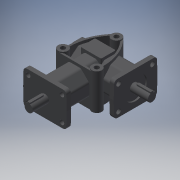
# Autodesk Inventor part: KBX-151L
Saved by Autodesk Inventor 2018 (Build 220112000, 112)
## iProperties
Category: PARTsolutions
Company: KHK
Created: 2017-10-24
Part Number: KBX-151L
Catalog Web Link: www.cadenas.de
Description: Bevel Box (KBXL)-
Vendor: KHK
Document SubType Name: Modeling
Designer: psAdmin
Manufacturer: KHK
Mass: 507.667 g
Surface Area: 746.565 cm^2
Volume: 507.667 cm^3
Density: 1 g/cm^3
Material: 一般
Appearance: PSOLRGB-175-175-175
PSOL_IDENT_0: {$CADENAS_DATA\23d-libs\khk\other_products\bevel_box_kbxl.prj},168 {VTYP=3D},{NB=KBX-151L},{LINA=KBX
PSOL_IDENT_1: -151L},{NN=Bevel Box (KBXL)},{DATE=08.02.2017 09:55:25},{GEOMDATE=11.03.2010 06:12:00},{VERSION=},{L
PSOL_IDENT_2: INEID=40},{LINESUBID=-1},{WBVAR=}  {NB=KBX-151L},{LINA=KBX-151L},{KT=DUMMY},{CN=KBX-151L},{SR=1:1},{
PSOL_IDENT_3: A=66},{B=100},{C=31},{D=36},{E=31},{F=22},{G=80},{H=62},{I=66},{J=140},{K=8},{L=137},{M=170},{P=30},
PSOL_IDENT_4: {Q=8.5},{R=8.5},{S=15},{T=42},{U=3},{KEY=5×5×27L},{WMF=LBX01.WMF},{Q1=8.5},{R1=8.5},{S1=15},{T1=42},
PSOL_IDENT_5: {R11=6},{R12=4.25},{F1=9.5},{F11=5},{F12=27},{E1=52},{E1R=6},{E11=46},{E11R=5},{RGX=57.275},{RGY=73.
PSOL_IDENT_6: 724},{RG1=90},{RG2=86.5},{RG3=9.01},{PLX=38},{PLY=27},{PL=16.23}
NN: Bevel Box (KBXL)
NB: KBX-151L
NBSYN: $CN.
LINA: KBX-151L
CN: KBX-151L
SR: 1:1
A: 66
B: 100
C: 31
D: 36
E: 31
F: 22
G: 80
H: 62
I: 66
J: 140
K: 8
L: 137
M: 170
P: 30
Q: 8.5
R: 8.5
S: 15
T: 42
U: 3
KEY: 5x5x27L
SUPPLIER: KHK
ARTICLENO: KBX-151L
BOMINFO: KBX-151L
CREATOR: CADENAS GmbH
Title: KBX-151L
Author: Cadenas PARTsolutions
Autodesk Inventor part; units mm, degrees
ref_plane "YZ Plane" through (0, 0, 0) normal (1, 0, 0) x (0, 1, 0)
ref_plane "XZ Plane" through (0, 0, 0) normal (0, 1, 0) x (-1, 0, 0)
ref_plane "XY Plane" through (0, 0, 0) normal (0, 0, 1) x (1, 0, 0)
sketch "Sketch_1" plane through (0, 0, 0) normal (0, 1, 0) x (1, 0, 0)
  line L0 (-40, 0) -> (-39.3412, -25.1571)
  arc A0 (-39.3412, -25.1571) -> (-33.3433, -31) centre (-33.3433, -25) ccw
  line L1 (-33.3433, -31) -> (33.3433, -31)
  arc A1 (33.3433, -31) -> (39.3412, -25.1571) centre (33.3433, -25) ccw
  line L2 (39.3412, -25.1571) -> (40, 0)
  line L3 (40, 0) -> (39.3412, 25.1571)
  arc A2 (39.3412, 25.1571) -> (33.3433, 31) centre (33.3433, 25) ccw
  line L4 (33.3433, 31) -> (-33.3433, 31)
  arc A3 (-33.3433, 31) -> (-39.3412, 25.1571) centre (-33.3433, 25) ccw
  line L5 (-39.3412, 25.1571) -> (-40, 0)
  circle A4 centre (31, 22) radius 4.25
  circle A5 centre (31, -22) radius 4.25
  circle A6 centre (-31, 22) radius 4.25
  circle A7 centre (-31, -22) radius 4.25
  constraints: 12 end point, 8 centre point, 8 point on circle
extrude "Extrusion1" add sketch "Sketch_1" along normal blind 8
sketch "Sketch2" plane through (0, 0, 0) normal (0, -1, 0) x (1, 0, 0)
  point P0 (0, 0)
hole "Hole1" at (0, 0, 0) direction (0, 1, 0) diameter 42 depth 3
sketch "Sketch_3" plane through (0, 0, 0) normal (0, 0, 1) x (1, 0, 0)
  line L0 (0, -30) -> (0, 8)
  line L1 (0, 8) -> (7.5, 8)
  line L2 (7.5, 8) -> (7.5, -30)
  line L3 (7.5, -30) -> (0, -30)
  line L4 (0, -30) -> (0, 8)
  constraints: 10 end point
revolve "Revolution1" add sketch "Sketch_3" angle 360 about axis through (0, -30, 0) along (0, -1, 0)
sketch "Sketch_5" plane through (0, 0, 0) normal (0, 0, 1) x (1, 0, 0)
  line L0 (-2.5, -5.5) -> (-2.5, -30)
  line L1 (-2.5, -30) -> (2.5, -30)
  line L2 (2.5, -30) -> (2.5, -5.5)
  arc A0 (2.5, -5.5) -> (-2.5, -5.5) centre (0, -5.5) ccw
  constraints: 6 end point, 2 point on circle, 1 centre point
extrude "Extrusion2" add sketch "Sketch_5" along normal blind 9.5
sketch "Sketch_6" plane through (0, 0, 0) normal (0, 1, 0) x (1, 0, 0)
  line L0 (-26, 8.2843) -> (-26, -8.2843)
  arc A0 (-26, -8.2843) -> (-24.2426, -12.5269) centre (-20, -8.2843) ccw
  line L1 (-24.2426, -12.5269) -> (-12.5269, -24.2426)
  arc A1 (-12.5269, -24.2426) -> (-8.2843, -26) centre (-8.2843, -20) ccw
  line L2 (-8.2843, -26) -> (8.2843, -26)
  arc A2 (8.2843, -26) -> (12.5269, -24.2426) centre (8.2843, -20) ccw
  line L3 (12.5269, -24.2426) -> (24.2426, -12.5269)
  arc A3 (24.2426, -12.5269) -> (26, -8.2843) centre (20, -8.2843) ccw
  line L4 (26, -8.2843) -> (26, 8.2843)
  arc A4 (26, 8.2843) -> (24.2426, 12.5269) centre (20, 8.2843) ccw
  line L5 (24.2426, 12.5269) -> (12.5269, 24.2426)
  arc A5 (12.5269, 24.2426) -> (8.2843, 26) centre (8.2843, 20) ccw
  line L6 (8.2843, 26) -> (-8.2843, 26)
  arc A6 (-8.2843, 26) -> (-12.5269, 24.2426) centre (-8.2843, 20) ccw
  line L7 (-12.5269, 24.2426) -> (-24.2426, 12.5269)
  arc A7 (-24.2426, 12.5269) -> (-26, 8.2843) centre (-20, 8.2843) ccw
  constraints: 16 end point, 16 point on circle, 8 centre point
extrude "Extrusion3" add sketch "Sketch_6" along normal blind 100
sketch "Sketch_7" plane through (0, 0, 0) normal (1, 0, 0) x (0, 0, -1)
  line L0 (-26, 108.2843) -> (-26, 91.7157)
  arc A0 (-26, 91.7157) -> (-24.2426, 87.4731) centre (-20, 91.7157) ccw
  line L1 (-24.2426, 87.4731) -> (-12.5269, 75.7574)
  arc A1 (-12.5269, 75.7574) -> (-8.2843, 74) centre (-8.2843, 80) ccw
  line L2 (-8.2843, 74) -> (8.2843, 74)
  arc A2 (8.2843, 74) -> (12.5269, 75.7574) centre (8.2843, 80) ccw
  line L3 (12.5269, 75.7574) -> (24.2426, 87.4731)
  arc A3 (24.2426, 87.4731) -> (26, 91.7157) centre (20, 91.7157) ccw
  line L4 (26, 91.7157) -> (26, 108.2843)
  arc A4 (26, 108.2843) -> (24.2426, 112.5269) centre (20, 108.2843) ccw
  line L5 (24.2426, 112.5269) -> (12.5269, 124.2426)
  arc A5 (12.5269, 124.2426) -> (8.2843, 126) centre (8.2843, 120) ccw
  line L6 (8.2843, 126) -> (-8.2843, 126)
  arc A6 (-8.2843, 126) -> (-12.5269, 124.2426) centre (-8.2843, 120) ccw
  line L7 (-12.5269, 124.2426) -> (-24.2426, 112.5269)
  arc A7 (-24.2426, 112.5269) -> (-26, 108.2843) centre (-20, 108.2843) ccw
  constraints: 16 end point, 16 point on circle, 8 centre point
extrude "Extrusion4" add sketch "Sketch_7" along normal mid plane 132
sketch "Sketch_9" plane through (0, 0, 0) normal (0, 0, 1) x (1, 0, 0)
  line L0 (-71, 69) -> (-31.5995, 69)
  arc A0 (-10.8459, 131) -> (-31.5995, 69) centre (57.275, 73.724) ccw
  line L1 (-10.8459, 131) -> (-71, 131)
  line L2 (-71, 131) -> (-71, 69)
  constraints: 6 end point, 2 point on circle, 1 centre point
extrude "Extrusion5" cut sketch "Sketch_9" along normal mid plane 80
sketch "Sketch_10" plane through (0, 0, 0) normal (1, 0, 0) x (0, 0, -1)
  line L0 (-23, 107.4558) -> (-23, 92.5442)
  arc A0 (-23, 92.5442) -> (-21.5355, 89.0086) centre (-18, 92.5442) ccw
  line L1 (-21.5355, 89.0086) -> (-10.9914, 78.4645)
  arc A1 (-10.9914, 78.4645) -> (-7.4558, 77) centre (-7.4558, 82) ccw
  line L2 (-7.4558, 77) -> (7.4558, 77)
  arc A2 (7.4558, 77) -> (10.9914, 78.4645) centre (7.4558, 82) ccw
  line L3 (10.9914, 78.4645) -> (21.5355, 89.0086)
  arc A3 (21.5355, 89.0086) -> (23, 92.5442) centre (18, 92.5442) ccw
  line L4 (23, 92.5442) -> (23, 107.4558)
  arc A4 (23, 107.4558) -> (21.5355, 110.9914) centre (18, 107.4558) ccw
  line L5 (21.5355, 110.9914) -> (10.9914, 121.5355)
  arc A5 (10.9914, 121.5355) -> (7.4558, 123) centre (7.4558, 118) ccw
  line L6 (7.4558, 123) -> (-7.4558, 123)
  arc A6 (-7.4558, 123) -> (-10.9914, 121.5355) centre (-7.4558, 118) ccw
  line L7 (-10.9914, 121.5355) -> (-21.5355, 110.9914)
  arc A7 (-21.5355, 110.9914) -> (-23, 107.4558) centre (-18, 107.4558) ccw
  constraints: 16 end point, 16 point on circle, 8 centre point
extrude "Extrusion6" add sketch "Sketch_10" against normal blind 41
sketch "Sketch_11" plane through (0, 0, 0) normal (0, 0, 1) x (1, 0, 0)
  arc A0 (-19, 85.77) -> (-17, 83.77) centre (-17, 85.77) ccw
  line L0 (-17, 83.77) -> (17, 83.77)
  arc A1 (17, 83.77) -> (19, 85.77) centre (17, 85.77) ccw
  line L1 (19, 85.77) -> (19, 108.77)
  arc A2 (19, 108.77) -> (17, 110.77) centre (17, 108.77) ccw
  line L2 (17, 110.77) -> (-17, 110.77)
  arc A3 (-17, 110.77) -> (-19, 108.77) centre (-17, 108.77) ccw
  line L3 (-19, 108.77) -> (-19, 85.77)
  constraints: 8 end point, 8 point on circle, 4 centre point
extrude "Extrusion7" add sketch "Sketch_11" along normal blind 31
sketch "Sketch_12" plane through (0, 0, 0) normal (0, 0, 1) x (1, 0, 0)
  arc A0 (-32.7207, 72.8442) -> (-31, 54.99) centre (-31, 64) ccw
  line L0 (-31, 54.99) -> (31, 54.99)
  arc A1 (31, 54.99) -> (32.7207, 72.8442) centre (31, 64) ccw
  arc A2 (32.7207, 72.8442) -> (6.6762, 137.0504) centre (-57.275, 73.724) ccw
  arc A3 (6.6762, 137.0504) -> (-6.0503, 137.6764) centre (0, 131) ccw
  arc A4 (-6.0503, 137.6764) -> (-32.7207, 72.8442) centre (57.275, 73.724) ccw
  arc A5 (-8.8769, 129.4571) -> (-29.2204, 72.8325) centre (57.275, 73.724) ccw
  arc A6 (-23.8712, 58.49) -> (-29.2204, 72.8325) centre (-31, 64) ccw
  line L1 (-23.8712, 58.49) -> (23.8712, 58.49)
  arc A7 (29.2204, 72.8325) -> (23.8712, 58.49) centre (31, 64) ccw
  arc A8 (29.2204, 72.8325) -> (8.8769, 129.4571) centre (-57.275, 73.724) ccw
  arc A9 (-8.8769, 129.4571) -> (8.8769, 129.4571) centre (0, 131) ccw
  constraints: 20 point on circle, 10 centre point, 4 end point
extrude "Extrusion8" add sketch "Sketch_12" along normal mid plane 62
sketch "Sketch_21" plane through (0, 0, 0) normal (0, 0, 1) x (1, 0, 0)
  circle A0 centre (0, 131) radius 9.01
  constraints: 1 centre point
extrude "Extrusion9" add sketch "Sketch_21" along normal mid plane 66
sketch "Sketch_13" plane through (0, 0, 0) normal (0, 0, 1) x (1, 0, 0)
  circle A0 centre (0, 131) radius 4.25
  constraints: 1 centre point
extrude "Extrusion10" cut sketch "Sketch_13" along normal mid plane 66
sketch "Sketch_22" plane through (0, 0, 0) normal (0, 0, 1) x (1, 0, 0)
  circle A0 centre (31, 64) radius 9.01
  constraints: 1 centre point
extrude "Extrusion11" add sketch "Sketch_22" along normal mid plane 66
sketch "Sketch_14" plane through (0, 0, 0) normal (0, 0, 1) x (1, 0, 0)
  circle A0 centre (31, 64) radius 4.25
  constraints: 1 centre point
extrude "Extrusion12" cut sketch "Sketch_14" along normal mid plane 66
sketch "Sketch_23" plane through (0, 0, 0) normal (0, 0, 1) x (1, 0, 0)
  circle A0 centre (-31, 64) radius 9.01
  constraints: 1 centre point
extrude "Extrusion13" add sketch "Sketch_23" along normal mid plane 66
sketch "Sketch_15" plane through (0, 0, 0) normal (0, 0, 1) x (1, 0, 0)
  circle A0 centre (-31, 64) radius 4.25
  constraints: 1 centre point
extrude "Extrusion14" cut sketch "Sketch_15" along normal mid plane 66
sketch "Sketch_16" plane through (66, 0, 0) normal (1, 0, 0) x (0, 0, -1)
  line L0 (-31, 133.3433) -> (-31, 66.6567)
  arc A0 (-31, 66.6567) -> (-25.1571, 60.6588) centre (-25, 66.6567) ccw
  line L1 (-25.1571, 60.6588) -> (0, 60)
  line L2 (0, 60) -> (25.1571, 60.6588)
  arc A1 (25.1571, 60.6588) -> (31, 66.6567) centre (25, 66.6567) ccw
  line L3 (31, 66.6567) -> (31, 133.3433)
  arc A2 (31, 133.3433) -> (25.1571, 139.3412) centre (25, 133.3433) ccw
  line L4 (25.1571, 139.3412) -> (0, 140)
  line L5 (0, 140) -> (-25.1571, 139.3412)
  arc A3 (-25.1571, 139.3412) -> (-31, 133.3433) centre (-25, 133.3433) ccw
  circle A4 centre (22, 69) radius 4.25
  circle A5 centre (22, 131) radius 4.25
  circle A6 centre (-22, 69) radius 4.25
  circle A7 centre (-22, 131) radius 4.25
  constraints: 12 end point, 8 centre point, 8 point on circle
extrude "Extrusion15" add sketch "Sketch_16" against normal blind 8
sketch "Sketch18" plane through (66, 0, 0) normal (1, 0, 0) x (0, 0, -1)
  point P0 (0, 100)
hole "Hole2" at (66, 100, 0) direction (-1, 0, 0) diameter 42 depth 3
sketch "Sketch_18" plane through (66, 0, 0) normal (1, 0, 0) x (0, 0, -1)
  circle A0 centre (0, 100) radius 7.5
  constraints: 1 centre point
extrude "Extrusion16" add sketch "Sketch_18" along normal mid plane 60
sketch "Sketch_20" plane through (0, 0, 0) normal (0, 0, 1) x (1, 0, 0)
  arc A0 (71.5, 102.5) -> (71.5, 97.5) centre (71.5, 100) ccw
  line L0 (71.5, 97.5) -> (96, 97.5)
  line L1 (96, 97.5) -> (96, 102.5)
  line L2 (96, 102.5) -> (71.5, 102.5)
  constraints: 6 end point, 2 point on circle, 1 centre point
extrude "Extrusion17" add sketch "Sketch_20" along normal blind 9.5
body "Solid1"
